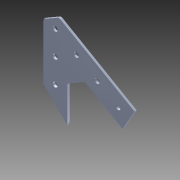
# Autodesk Inventor part: Versaframe 60deg gusset
Saved by Autodesk Inventor 2015 SP1 (Build 190203100, 203)
## iProperties
Created: 2015-01-17
Part Number: Versaframe 60deg gusset
Material: Aluminum 6061
Document SubType Name: Modeling
Designer: Jarod
Density: 2.7 g/cm^3
Appearance: Aluminum - Flat
Title: 217-3551-STEP.STEP
Description: STEP AP214
Creation Date: 2013-12-10
Sending System: SolidWorks 2013
Preprocessor: SwSTEP 2.0
Author: Jarod
Autodesk Inventor part; units mm, degrees
ref_plane "YZ Plane" through (0, 0, 0) normal (1, 0, 0) x (0, 1, 0)
ref_plane "XZ Plane" through (0, 0, 0) normal (0, 1, 0) x (-1, 0, 0)
ref_plane "XY Plane" through (0, 0, 0) normal (0, 0, 1) x (1, 0, 0)
sketch "Sketch3" plane through (-10.4876, -69.85, 2.286) normal (0, -1, 0) x (1, 0, 0)
  line L0 (0, 0) -> (22.7558, 0) projected
  line L1 (0, -2.286) -> (0, 0) projected
  line L2 (0, -2.286) -> (22.7558, -2.286) projected
  line L3 (22.7558, -2.286) -> (22.7558, 0) projected
  line L4 (22.7558, 0) -> (23.3146, 0) projected
  line L5 (22.7558, -2.286) -> (22.7558, 0) projected
  line L6 (22.7558, -2.286) -> (23.3146, -2.286) projected
  line L7 (23.3146, -2.286) -> (23.3146, 0) projected
  line L8 (0, 0) -> (-2.0854, 0) projected
  line L9 (-2.0854, -2.286) -> (-2.0854, 0) projected
  line L10 (0, -2.286) -> (-2.0854, -2.286) projected
  line L11 (0, -2.286) -> (0, 0) projected
  point P0 (10.4876, -2.286)
extrude "Extrusion3" add sketch "Sketch3" along normal mid plane 38.1
sketch "Sketch4" plane through (65.7357, -25.8425, 2.286) normal (0.866, -0.5, 0) x (0, 0, -1)
  line L0 (2.286, 0) -> (0, 0) projected
  line L1 (0, -22.7558) -> (0, 0) projected
  line L2 (2.286, -22.7558) -> (0, -22.7558) projected
  line L3 (2.286, -22.7558) -> (2.286, 0) projected
  line L4 (0, 0) -> (0, 2.0854) projected
  line L5 (2.286, 0) -> (0, 0) projected
  line L6 (2.286, 0) -> (2.286, 2.0854) projected
  line L7 (2.286, 2.0854) -> (0, 2.0854) projected
  line L8 (0, -23.3146) -> (0, -22.7558) projected
  line L9 (2.286, -23.3146) -> (0, -23.3146) projected
  line L10 (2.286, -23.3146) -> (2.286, -22.7558) projected
  line L11 (2.286, -22.7558) -> (0, -22.7558) projected
  point P0 (2.286, -10.4876)
extrude "Extrusion4" add sketch "Sketch4" along normal mid plane 38.1
sketch "Sketch5" plane through (12.827, -88.9, 0) normal (0, 0, -1) x (-1, 0, 0)
  arc A0 (-30.132, 61.7072) -> (-32.2021, 65.2928) centre (-31.1671, 63.5) ccw projected
  line L0 (-32.2021, 65.2928) -> (-30.132, 61.7072) projected
  line L1 (7.3756, 100.2707) -> (-70.4492, 55.3385) projected
  line L2 (-57.7492, 33.3415) -> (-70.4492, 55.3385) projected
  line L3 (-4.7625, 63.9334) -> (-57.7492, 33.3415) projected
  arc A1 (0, 61.1837) -> (-4.7625, 63.9334) centre (-3.175, 61.1837) ccw projected
  line L4 (0, 61.1837) -> (0, 0) projected
  line L5 (25.4, 0) -> (0, 0) projected
  line L6 (25.4, 89.8643) -> (25.4, 0) projected
  line L7 (24.8412, 91.9497) -> (25.4, 89.8643) projected
  line L8 (9.461, 100.8295) -> (24.8412, 91.9497) projected
  line L9 (9.461, 100.8295) -> (7.3756, 100.2707) projected
  arc A2 (14.8971, 38.1) -> (10.7569, 38.1) centre (12.827, 38.1) ccw projected
  line L10 (10.7569, 38.1) -> (14.8971, 38.1) projected
  circle A3 centre (-9.17, 76.2) radius 2.0701 projected
  circle A4 centre (12.827, 88.9) radius 2.0701 projected
  circle A5 centre (12.827, 63.5) radius 2.0701 projected
extrude "Extrusion5" add sketch "Sketch5" against normal blind 2.286
sketch "Sketch6" plane through (12.827, -88.9, 0) normal (0, 0, -1) x (-1, 0, 0)
  arc A0 (-30.132, 61.7072) -> (-32.2021, 65.2928) centre (-31.1671, 63.5) ccw projected
  line L0 (-57.7492, 33.3415) -> (-70.4492, 55.3385) projected
  line L1 (-4.7625, 63.9334) -> (-57.7492, 33.3415) projected
  line L2 (25.4, 89.8643) -> (25.4, 0) projected
  arc A1 (14.8971, 38.1) -> (10.7569, 38.1) centre (12.827, 38.1) ccw projected
  circle A2 centre (-9.17, 76.2) radius 2.0701 projected
  circle A3 centre (12.827, 88.9) radius 2.0701 projected
  circle A4 centre (12.827, 63.5) radius 2.0701 projected
  circle A5 centre (12.827, 88.9) radius 2.54
  circle A6 centre (-9.17, 76.2) radius 2.54
  circle A7 centre (12.827, 63.5) radius 2.54
  circle A8 centre (12.827, 38.1) radius 2.54
  circle A9 centre (-31.1671, 63.5) radius 2.54
  circle A10 centre (-53.1006, 50.69) radius 2.54
  circle A11 centre (12.7, 12.7) radius 2.54
  dimension "d20" = 5.08
  dimension "d21" = 5.08
  dimension "d22" = 5.08
  dimension "d23" = 5.08
  dimension "d24" = 5.08
  dimension "d25" = 5.08
  dimension "d26" = 5.08
  dimension "d27" = 12.7
  dimension "d28" = 25.4
  dimension "d29" = 12.7
  dimension "d30" = 12.7
  constraints: 7 centre point, 5 coincident
  measures "d20" diameter of A5
  measures "d21" diameter of A6
  measures "d22" diameter of A7
  measures "d23" diameter of A8
  measures "d24" diameter of A9
  measures "d25" diameter of A10
  measures "d26" diameter of A11
  measures "d27" distance from line of L2 A11.centre
  measures "d28" vertical distance of A1.centre A11.centre
  measures "d29" distance from line of L1 A10.centre
  measures "d30" distance from line of L0 A10.centre
extrude "Extrusion6" cut sketch "Sketch6" against normal blind 2.286 contours A2 | A3 | A4 | A5 | A6 | A7 | A8 | A9 | A10 | A11
sketch "Sketch7" plane through (12.827, -88.9, 0) normal (0, 0, -1) x (-1, 0, 0)
  circle A0 centre (12.827, 38.1) radius 2.54 projected
  circle A1 centre (-31.1671, 63.5) radius 2.54 projected
  line L0 (-4.7625, 63.9334) -> (-57.7492, 33.3415) projected
  arc A2 (0, 61.1837) -> (-4.7625, 63.9334) centre (-3.175, 61.1837) ccw projected
  line L1 (0, 61.1837) -> (0, 0) projected
  line L2 (-31.1671, 63.5) -> (12.827, 38.1) construction
  line L3 (-18.3401, 56.0943) -> (0, 66.683)
  line L4 (0, 66.683) -> (0, 45.5057)
  line L5 (0, 61.1837) -> (0, 0) projected
  line L6 (0, 45.5057) -> (-18.3401, 56.0943)
  constraints: 8 end point, 6 point on line, 1 collinear
extrude "Extrusion7" add sketch "Sketch7" against normal blind 2.286 contours A2 L1 L6 L0
